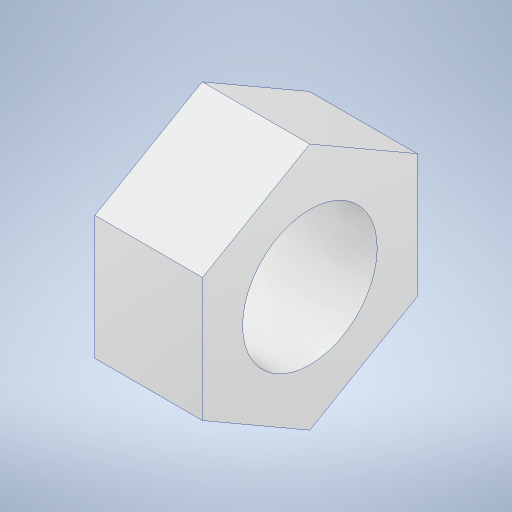
# Autodesk Inventor part: 5min-nut
Saved by Autodesk Inventor 2024.1 (Build 281209000, 209)
## iProperties
Created: 2023-10-01
Part Number: 5min-nut
Material: アルミニウム 6061
Document SubType Name: Modeling
Designer: haruy
Density: 2.7 g/cm^3
Appearance: アルミニウム - フラット
Author: haruy
Autodesk Inventor part; units mm, degrees
ref_plane "YZ Plane" through (0, 0, 0) normal (1, 0, 0) x (0, 1, 0)
ref_plane "XZ Plane" through (0, 0, 0) normal (0, 1, 0) x (-1, 0, 0)
ref_plane "XY Plane" through (0, 0, 0) normal (0, 0, 1) x (1, 0, 0)
sketch "スケッチ1" plane through (0, 0, 0) normal (1, 0, 0) x (0, 1, 0)
  circle A0 centre (0, 0) radius 4.6
  line L0 (4.6, 0) -> (2.3, 3.9837)
  line L1 (2.3, 3.9837) -> (-2.3, 3.9837)
  line L2 (-2.3, 3.9837) -> (-4.6, 0)
  line L3 (-4.6, 0) -> (-2.3, -3.9837)
  line L4 (2.3, -3.9837) -> (-2.3, -3.9837)
  line L5 (2.3, -3.9837) -> (4.6, 0)
  circle A1 centre (0, 0) radius 2.5
  point P0 (-2.3, -3.9837)
  dimension "d0" = 9.2
  dimension "d3" = 360
  dimension "d5" = 5
  constraints: 12 end point, 3 parallel, 3 point on circle, 2 centre point, 2 coincident, 1 horizontal, 7 other
  measures "d0" diameter of A0
  measures "d5" diameter of A1
extrude "押し出し1" add sketch "スケッチ1" along normal blind 4 contours L5 L4 L3 L2 L1 L0
